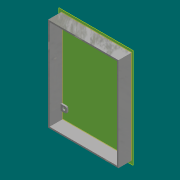
# Autodesk Inventor part: Struttura
Saved by Autodesk Inventor 2020 (Build 240168000, 168)
## iProperties
Created: 2025-01-02
Part Number: Struttura
Material: Plastica ABS
Document SubType Name: Modeling
Designer: Nicola Milia
Density: 1.06 g/cm^3
Appearance: Liscia - Bianco
Author: Nicola Milia
Autodesk Inventor part; units mm, degrees
ref_plane "YZ Plane" through (0, 0, 0) normal (1, 0, 0) x (0, 1, 0)
ref_plane "XZ Plane" through (0, 0, 0) normal (0, 1, 0) x (-1, 0, 0)
ref_plane "XY Plane" through (0, 0, 0) normal (0, 0, 1) x (1, 0, 0)
sketch "Schizzo1" plane through (0, 0, 0) normal (0, 0, 1) x (1, 0, 0)
  point P0 (0, 0)
sketch "Schizzo2" plane through (0, 0, 0) normal (0, 0, 1) x (1, 0, 0)
  line L0 (0, -121) -> (90, -121) projected
  line L1 (90, -121) -> (90, 0) projected
  line L2 (0, 0) -> (0, -121) projected
  line L3 (90, 0) -> (0, 0) projected
  circle A0 centre (86, -106) radius 2 projected
  circle A1 centre (4, -106) radius 2 projected
  circle A2 centre (4, -6) radius 2 projected
  circle A3 centre (86, -6) radius 2 projected
  line L4 (92, 2) -> (92, -123)
  line L5 (92, -123) -> (-2, -123)
  line L6 (-2, -123) -> (-2, 2)
  line L7 (-2, 2) -> (92, 2)
  dimension "d0" = 2
  constraints: 8 end point, 3 other
  measures "d0" distance between parallel lines of L1 L4
extrude "Estrusione1" add sketch "Schizzo2" along normal blind 18 contours L4 L5 L6 L7
ref_plane "Piano di lavoro1" through (45, -60.5, 1) normal (0, 0, 1) x (1, 0, 0)
sketch "Schizzo3" plane through (45, -60.5, 1) normal (0, 0, 1) x (1, 0, 0)
  circle A0 centre (41, -45.5) radius 2 projected
  circle A1 centre (-41, -45.5) radius 2 projected
  circle A2 centre (41, 54.5) radius 2 projected
  circle A3 centre (-41, 54.5) radius 2 projected
  line L0 (45, -60.5) -> (45, 60.5) projected
  line L1 (45, 60.5) -> (-45, 60.5) projected
  line L2 (-45, -60.5) -> (45, -60.5) projected
  line L3 (-45, 60.5) -> (-45, -60.5) projected
  line L4 (-45, -60.5) -> (-45, 60.5) projected
  line L5 (-39, -41.5) -> (-45, -41.5)
  line L6 (-45, -41.5) -> (-45, -49.5)
  line L7 (-45, -49.5) -> (-39, -49.5)
  line L8 (-37, -47.5) -> (-37, -43.5)
  arc A4 (-37, -43.5) -> (-39, -41.5) centre (-39, -43.5) ccw
  arc A5 (-39, -49.5) -> (-37, -47.5) centre (-39, -47.5) ccw
  line L9 (39, -41.5) -> (45, -41.5)
  line L10 (45, -41.5) -> (45, -49.5)
  line L11 (45, -49.5) -> (39, -49.5)
  line L12 (37, -47.5) -> (37, -43.5)
  arc A6 (37, -47.5) -> (39, -49.5) centre (39, -47.5) ccw
  arc A7 (39, -41.5) -> (37, -43.5) centre (39, -43.5) ccw
  line L13 (37, 60.5) -> (37, 52.5)
  line L14 (39, 50.5) -> (45, 50.5)
  line L15 (45, 50.5) -> (45, 60.5)
  arc A8 (37, 52.5) -> (39, 50.5) centre (39, 52.5) ccw
  line L16 (-45, 60.5) -> (-45, 50.5)
  line L17 (-45, 50.5) -> (-37, 50.5)
  line L18 (-37, 50.5) -> (-37, 60.5)
  point P0 (-45, -41.5)
  point P1 (-45, -49.5)
  point P2 (45, 50.5)
  constraints: 28 end point, 10 point on circle, 10 tangent, 6 parallel, 5 centre point, 4 perpendicular, 4 point on line, 2 equal radius
extrude "Estrusione2" add sketch "Schizzo3" along normal blind 2 contours L11 A6 L12 A7 L9 L0 | L3 L5 A4 L8 A5 L7 | L14 A8 L13 L1 L0 | L3 L1 L18 L17
fillet "Raccordo1" radius 2 1 edges at (8, -10, 2)
